Autodesk Fusion 360 part; units mm, degrees
(part 3 of 11)
  line L1668 (14.4479, -219.9183) -> (14.483, -219.9371)
  arc A104 (18.4614, -173.1211) -> (18.12, -173.2625) centre (18.32, -173.2625) ccw
  arc A105 (13.1828, -218.1997) -> (13.0414, -218.5411) centre (13.1828, -218.3997) ccw
  line L1669 (0.0013, -74.5276) -> (-0.0174, -74.5626)
  line L1670 (18.12, -173.2625) -> (18.12, -175.4997)
  line L1671 (6.2199, -29.9997) -> (6.02, -30.1995)
  line L1672 (-0.0787, -74.7914) -> (-0.08, -74.8997)
  line L1673 (0.0706, -74.4308) -> (0.0454, -74.4616)
  line L1674 (6.02, -29.7998) -> (6.2199, -29.9997)
  line L1675 (19.9148, -174.7519) -> (19.9083, -174.7127)
  line L1676 (-0.08, -74.8997) -> (-0.08, -78.4997)
  line L1677 (0.0454, -74.4616) -> (0.0223, -74.4938)
  line L1678 (-0.0338, -34.5988) -> (-0.0478, -34.636)
  line L1679 (14.3819, -219.8742) -> (14.4142, -219.8974)
  line L1680 (19.8738, -174.5988) -> (19.8574, -174.5626)
  line L1681 (6.02, -27.1603) -> (6.02, -29.7998)
  line L1682 (-0.0478, -74.636) -> (-0.0593, -74.674)
  line L1683 (19.8993, -174.674) -> (19.8878, -174.636)
  line L1684 (14.5943, -219.979) -> (14.633, -219.988)
  line L1685 (19.7946, -174.4616) -> (19.7694, -174.4308)
  line L1686 (14.3512, -219.849) -> (14.3819, -219.8742)
  line L1687 (6.02, -30.1995) -> (6.02, -32.839)
  line L1688 (-0.0683, -74.7127) -> (-0.0748, -74.7519)
  line L1689 (18.12, -175.4997) -> (16.4807, -175.4997)
  line L1690 (16.4807, -175.4997) -> (13.82, -172.839)
  line L1691 (3.6807, -37.2997) -> (7.0807, -33.8997)
  line L1692 (16.1593, -162.6997) -> (12.7593, -166.0997)
  line L1693 (7.0807, -173.8997) -> (9.713, -173.8997)
  line L1694 (9.92, -33.6927) -> (10.127, -33.8997)
  circle A106 centre (9.92, -29.9997) radius 2.1
  line L1695 (19.8177, -214.4938) -> (19.7946, -214.4616)
  arc A107 (1.72, -73.2625) -> (1.3786, -73.1211) centre (1.52, -73.2625) ccw
  line L1696 (18.12, -215.4997) -> (16.4807, -215.4997)
  line L1697 (-0.0593, -74.674) -> (-0.0683, -74.7127)
  arc A108 (1.72, -73.2625) -> (1.3786, -73.1211) centre (1.52, -73.2625) ccw
  line L1698 (19.8387, -214.5276) -> (19.8177, -214.4938)
  line L1699 (-0.0338, -74.5988) -> (-0.0478, -74.636)
  line L1700 (-0.0478, -74.636) -> (-0.0593, -74.674)
  line L1701 (14.483, -219.9371) -> (14.5191, -219.9534)
  line L1702 (16.1593, -162.6997) -> (12.7593, -166.0997)
  line L1703 (13.82, -167.1603) -> (16.4807, -164.4997)
  line L1704 (9.713, -166.0997) -> (7.0807, -166.0997)
  line L1705 (19.8387, -174.5276) -> (19.8177, -174.4938)
  line L1706 (16.4807, -175.4997) -> (13.82, -172.839)
  line L1707 (9.713, -33.8997) -> (9.92, -33.6927)
  line L1708 (9.713, -166.0997) -> (7.0807, -166.0997)
  line L1709 (18.42, -219.9997) -> (19.42, -219.9997)
  line L1710 (6.02, -32.839) -> (3.3593, -35.4997)
  line L1711 (-0.0174, -74.5626) -> (-0.0338, -74.5988)
  line L1712 (3.6807, -37.2997) -> (7.0807, -33.8997)
  line L1713 (0.0454, -74.4616) -> (0.0223, -74.4938)
  line L1714 (1.72, -35.4997) -> (1.72, -33.2625)
  line L1715 (-0.0338, -74.5988) -> (-0.0478, -74.636)
  line L1716 (0.0706, -74.4308) -> (0.0454, -74.4616)
  line L1717 (19.9187, -214.7914) -> (19.9148, -214.7519)
  line L1718 (3.3593, -75.4997) -> (1.72, -75.4997)
  line L1719 (6.02, -32.839) -> (3.3593, -35.4997)
  line L1720 (15.42, -218.1997) -> (13.1828, -218.1997)
  line L1721 (19.9148, -174.7519) -> (19.9083, -174.7127)
  line L1722 (-0.0174, -74.5626) -> (-0.0338, -74.5988)
  line L1723 (-0.0683, -74.7127) -> (-0.0748, -74.7519)
  line L1724 (13.82, -167.1603) -> (16.4807, -164.4997)
  line L1725 (19.8574, -174.5626) -> (19.8387, -174.5276)
  line L1726 (-0.08, -74.8997) -> (-0.08, -78.4997)
  line L1727 (9.92, -33.6927) -> (10.127, -33.8997)
  line L1728 (13.82, -30.1995) -> (13.6201, -29.9997)
  line L1729 (6.02, -72.839) -> (3.3593, -75.4997)
  line L1730 (4.42, -78.1997) -> (4.42, -76.5603)
  line L1731 (13.82, -32.839) -> (13.82, -30.1995)
  line L1732 (7.0807, -173.8997) -> (9.713, -173.8997)
  line L1733 (19.9083, -174.7127) -> (19.8993, -174.674)
  line L1734 (15.42, -216.5603) -> (15.42, -218.1997)
  line L1735 (1.72, -75.4997) -> (1.72, -73.2625)
  line L1736 (13.82, -29.7998) -> (13.82, -27.1603)
  arc A109 (6.7986, -78.5411) -> (6.6572, -78.1997) centre (6.6572, -78.3997) ccw
  line L1737 (19.9083, -214.7127) -> (19.8993, -214.674)
  line L1738 (13.0414, -218.5411) -> (14.3222, -219.8219)
  line L1739 (0.0223, -74.4938) -> (0.0013, -74.5276)
  line L1740 (1.72, -35.4997) -> (1.72, -33.2625)
  line L1741 (-0.0748, -74.7519) -> (-0.0787, -74.7914)
  line L1742 (0.0978, -74.4019) -> (0.0706, -74.4308)
  line L1743 (14.483, -219.9371) -> (14.5191, -219.9534)
  line L1744 (10.127, -33.8997) -> (12.7593, -33.8997)
  line L1745 (6.02, -72.839) -> (3.3593, -75.4997)
  line L1746 (13.6201, -29.9997) -> (13.82, -29.7998)
  line L1747 (13.82, -30.1995) -> (13.6201, -29.9997)
  line L1748 (4.42, -76.5603) -> (7.0807, -73.8997)
  line L1749 (13.82, -32.839) -> (13.82, -30.1995)
  line L1750 (19.8878, -214.636) -> (19.8738, -214.5988)
  line L1751 (13.6201, -29.9997) -> (13.82, -29.7998)
  line L1752 (1.3786, -73.1211) -> (0.0978, -74.4019)
  line L1753 (-0.08, -78.4997) -> (-0.08, -79.4997)
  line L1754 (19.8738, -214.5988) -> (19.8574, -214.5626)
  line L1755 (19.7694, -214.4308) -> (19.7422, -214.4019)
  arc A110 (13.0414, -81.4582) -> (13.1828, -81.7997) centre (13.1828, -81.5997) ccw
  line L1756 (19.92, -214.8311) -> (19.9187, -214.7914)
  line L1757 (9.7152, -73.8997) -> (9.92, -73.6949)
  line L1758 (19.7694, -34.4308) -> (19.7422, -34.4019)
  line L1759 (-0.08, -78.4997) -> (-0.08, -79.4997)
  line L1760 (19.92, -214.8311) -> (19.9187, -214.7914)
  line L1761 (10.127, -73.8997) -> (12.7593, -73.8997)
  line L1762 (19.7946, -214.4616) -> (19.7694, -214.4308)
  line L1763 (19.8574, -214.5626) -> (19.8387, -214.5276)
  line L1764 (18.12, -35.4997) -> (16.4807, -35.4997)
  line L1765 (4.42, -76.5603) -> (7.0807, -73.8997)
  arc A111 (19.42, -219.9997) -> (19.92, -219.4997) centre (19.42, -219.4997) ccw
  line L1766 (19.92, -219.4997) -> (19.92, -218.4997)
  line L1767 (4.42, -78.1997) -> (4.42, -76.5603)
  line L1768 (19.92, -218.4997) -> (19.92, -214.8311)
  line L1769 (5.5178, -79.8219) -> (6.7986, -78.5411)
  line L1770 (19.9083, -214.7127) -> (19.8993, -214.674)
  line L1771 (19.8574, -214.5626) -> (19.8387, -214.5276)
  line L1772 (19.7946, -214.4616) -> (19.7694, -214.4308)
  line L1773 (9.92, -73.6949) -> (10.127, -73.8997)
  line L1774 (18.12, -37.2997) -> (18.12, -42.6997)
  line L1775 (6.6572, -78.1997) -> (4.42, -78.1997)
  line L1776 (19.7694, -214.4308) -> (19.7422, -214.4019)
  line L1777 (19.8738, -34.5988) -> (19.8574, -34.5626)
  line L1778 (18.42, -219.9997) -> (19.42, -219.9997)
  arc A112 (19.42, -219.9997) -> (19.92, -219.4997) centre (19.42, -219.4997) ccw
  line L1779 (19.9148, -214.7519) -> (19.9083, -214.7127)
  line L1780 (5.5178, -79.8219) -> (6.7986, -78.5411)
  line L1781 (10.127, -33.8997) -> (12.7593, -33.8997)
  line L1782 (19.8177, -214.4938) -> (19.7946, -214.4616)
  line L1783 (19.92, -218.4997) -> (19.92, -214.8311)
  line L1784 (19.8387, -214.5276) -> (19.8177, -214.4938)
  line L1785 (9.713, -33.8997) -> (9.92, -33.6927)
  line L1786 (1.72, -75.4997) -> (1.72, -73.2625)
  line L1787 (19.8993, -214.674) -> (19.8878, -214.636)
  circle A113 centre (9.92, -29.9997) radius 2.1
  line L1788 (10.127, -73.8997) -> (12.7593, -73.8997)
  line L1789 (13.82, -29.7998) -> (13.82, -27.1603)
  line L1790 (9.92, -73.6949) -> (10.127, -73.8997)
  line L1791 (6.6572, -78.1997) -> (4.42, -78.1997)
  line L1792 (3.3593, -75.4997) -> (1.72, -75.4997)
  line L1793 (18.12, -42.6997) -> (16.1593, -42.6997)
  line L1794 (18.12, -33.2625) -> (18.12, -35.4997)
  line L1795 (19.9083, -34.7127) -> (19.8993, -34.674)
  line L1796 (19.92, -219.4997) -> (19.92, -218.4997)
  arc A114 (6.7986, -78.5411) -> (6.6572, -78.1997) centre (6.6572, -78.3997) ccw
  line L1797 (9.7152, -73.8997) -> (9.92, -73.6949)
  line L1798 (18.12, -215.4997) -> (16.4807, -215.4997)
  arc A115 (13.1828, -78.1997) -> (13.0414, -78.5411) centre (13.1828, -78.3997) ccw
  line L1799 (19.92, -34.8997) -> (19.9187, -34.7914)
  line L1800 (1.3786, -73.1211) -> (0.0978, -74.4019)
  line L1801 (19.9187, -214.7914) -> (19.9148, -214.7519)
  arc A116 (18.4614, -33.1211) -> (18.12, -33.2625) centre (18.32, -33.2625) ccw
  line L1802 (19.8993, -214.674) -> (19.8878, -214.636)
  arc A117 (13.1828, -78.1997) -> (13.0414, -78.5411) centre (13.1828, -78.3997) ccw
  arc A118 (13.0414, -81.4582) -> (13.1828, -81.7997) centre (13.1828, -81.5997) ccw
  line L1803 (19.8738, -214.5988) -> (19.8574, -214.5626)
  line L1804 (19.9083, -34.7127) -> (19.8993, -34.674)
  line L1805 (19.8878, -214.636) -> (19.8738, -214.5988)
  line L1806 (16.1593, -37.2997) -> (18.12, -37.2997)
  line L1807 (19.8574, -34.5626) -> (19.8387, -34.5276)
  line L1808 (19.7422, -214.4019) -> (18.4614, -213.1211)
  line L1809 (14.7514, -219.9997) -> (18.42, -219.9997)
  line L1810 (19.9148, -214.7519) -> (19.9083, -214.7127)
  line L1811 (18.12, -213.2625) -> (18.12, -215.4997)
  line L1812 (16.4807, -215.4997) -> (13.82, -212.839)
  line L1813 (19.8177, -34.4938) -> (19.7946, -34.4616)
  line L1814 (19.8738, -34.5988) -> (19.8574, -34.5626)
  line L1815 (12.7593, -213.8997) -> (15.42, -216.5603)
  line L1816 (18.12, -42.6997) -> (16.1593, -42.6997)
  line L1817 (14.7514, -219.9997) -> (18.42, -219.9997)
  line L1818 (-0.0787, -5.2079) -> (-0.0748, -5.2474)
  line L1819 (0.0978, -5.5975) -> (1.3786, -6.8782)
  line L1820 (5.2457, -0.0203) -> (5.207, -0.0113)
  line L1821 (4.42, -3.439) -> (4.42, -1.7997)
  line L1822 (5.207, -0.0113) -> (5.1678, -0.0049)
  line L1823 (5.4888, -0.1503) -> (5.4581, -0.1251)
  line L1824 (4.42, -1.7997) -> (6.6572, -1.7997)
  line L1825 (-0.08, -1.4997) -> (-0.08, -5.0997)
  line L1826 (1.42, 0.0003) -> (0.42, 0.0003)
  arc A119 (6.6572, -1.7997) -> (6.7986, -1.4582) centre (6.6572, -1.5997) ccw
  line L1827 (1.72, -4.4997) -> (3.3593, -4.4997)
  line L1828 (-0.0787, -5.2079) -> (-0.0748, -5.2474)
  line L1829 (7.0807, -6.0997) -> (4.42, -3.439)
  line L1830 (5.357, -0.0623) -> (5.3209, -0.0459)
  line L1831 (5.1283, -0.001) -> (5.0886, 0.0003)
  line L1832 (5.0886, 0.0003) -> (1.42, 0.0003)
  line L1833 (5.4258, -0.102) -> (5.3921, -0.081)
  arc A120 (13.0414, -1.4582) -> (13.1828, -1.7997) centre (13.1828, -1.5997) ccw
  line L1834 (13.6201, -9.9997) -> (13.82, -9.7998)
  line L1835 (-0.08, -1.4997) -> (-0.08, -5.0997)
  line L1836 (9.92, -6.3044) -> (9.7152, -6.0997)
  line L1837 (6.7986, -1.4582) -> (5.5178, -0.1775)
  line L1838 (12.7593, -6.0997) -> (10.127, -6.0997)
  line L1839 (7.0807, -6.0997) -> (4.42, -3.439)
  line L1840 (-0.0683, -5.2866) -> (-0.0593, -5.3253)
  line L1841 (1.42, 0.0003) -> (0.42, 0.0003)
  line L1842 (9.92, -6.3044) -> (9.7152, -6.0997)
  line L1843 (5.2837, -0.0319) -> (5.2457, -0.0203)
  line L1844 (5.4581, -0.1251) -> (5.4258, -0.102)
  line L1845 (5.2457, -0.0203) -> (5.207, -0.0113)
  line L1846 (-0.08, -0.4997) -> (-0.08, -1.4997)
  line L1847 (3.3593, -4.4997) -> (6.02, -7.1603)
  line L1848 (5.207, -0.0113) -> (5.1678, -0.0049)
  arc A121 (0.42, 0.0003) -> (-0.08, -0.4997) centre (0.42, -0.4997) ccw
  line L1849 (5.5178, -0.1775) -> (5.4888, -0.1503)
  line L1850 (5.1678, -0.0049) -> (5.1283, -0.001)
  line L1851 (1.72, -6.7368) -> (1.72, -4.4997)
  line L1852 (5.4258, -0.102) -> (5.3921, -0.081)
  line L1853 (1.72, -6.7368) -> (1.72, -4.4997)
  line L1854 (-0.08, -0.4997) -> (-0.08, -1.4997)
  line L1855 (5.3921, -0.081) -> (5.357, -0.0623)
  line L1856 (3.3593, -4.4997) -> (6.02, -7.1603)
  arc A122 (0.42, 0.0003) -> (-0.08, -0.4997) centre (0.42, -0.4997) ccw
  line L1857 (-0.0593, -5.3253) -> (-0.0478, -5.3633)
  line L1858 (5.5178, -0.1775) -> (5.4888, -0.1503)
  line L1859 (4.42, -3.439) -> (4.42, -1.7997)
  line L1860 (5.2837, -0.0319) -> (5.2457, -0.0203)
  line L1861 (6.7986, -1.4582) -> (5.5178, -0.1775)
  line L1862 (5.3921, -0.081) -> (5.357, -0.0623)
  line L1863 (0.0454, -5.5378) -> (0.0706, -5.5685)
  line L1864 (0.0706, -5.5685) -> (0.0978, -5.5975)
  line L1865 (5.3209, -0.0459) -> (5.2837, -0.0319)
  arc A123 (6.6572, -1.7997) -> (6.7986, -1.4582) centre (6.6572, -1.5997) ccw
  line L1866 (5.3209, -0.0459) -> (5.2837, -0.0319)
  line L1867 (5.357, -0.0623) -> (5.3209, -0.0459)
  line L1868 (5.1678, -0.0049) -> (5.1283, -0.001)
  line L1869 (5.4581, -0.1251) -> (5.4258, -0.102)
  line L1870 (-0.08, -5.0997) -> (-0.0787, -5.2079)
  line L1871 (0.0978, -5.5975) -> (1.3786, -6.8782)
  line L1872 (5.0886, 0.0003) -> (1.42, 0.0003)
  line L1873 (5.4888, -0.1503) -> (5.4581, -0.1251)
  line L1874 (0.0978, -25.5975) -> (1.3786, -26.8782)
  line L1875 (5.1283, -0.001) -> (5.0886, 0.0003)
  line L1876 (4.42, -1.7997) -> (6.6572, -1.7997)
  line L1877 (14.7117, -80.001) -> (14.6722, -80.0049)
  line L1878 (7.0807, -33.8997) -> (9.713, -33.8997)
  arc A124 (19.42, -79.9997) -> (19.92, -79.4997) centre (19.42, -79.4997) ccw
  line L1879 (0.0223, -25.5055) -> (0.0454, -25.5378)
  line L1880 (14.5563, -80.0319) -> (14.5191, -80.0459)
  line L1881 (-0.08, -34.8997) -> (-0.08, -45.0997)
  line L1882 (19.92, -45.0997) -> (19.92, -34.8997)
  line L1883 (-0.0593, -25.3253) -> (-0.0478, -25.3633)
  line L1884 (14.633, -80.0113) -> (14.5943, -80.0203)
  line L1885 (7.0807, -46.0997) -> (3.6807, -42.6997)
  line L1886 (-0.0787, -25.2079) -> (-0.0748, -25.2474)
  line L1887 (14.633, -80.0113) -> (14.5943, -80.0203)
  line L1888 (19.92, -81.4997) -> (19.92, -80.4997)
  line L1889 (14.7117, -79.9984) -> (14.7514, -79.9997)
  line L1890 (14.633, -79.988) -> (14.6722, -79.9945)
  line L1891 (14.6722, -80.0049) -> (14.633, -80.0113)
  line L1892 (18.42, -79.9997) -> (19.42, -79.9997)
  arc A125 (19.92, -80.4997) -> (19.42, -79.9997) centre (19.42, -80.4997) ccw
  line L1893 (14.5943, -80.0203) -> (14.5563, -80.0319)
  line L1894 (1.72, -26.7368) -> (1.72, -24.4997)
  line L1895 (-0.0683, -25.2866) -> (-0.0593, -25.3253)
  line L1896 (18.42, -79.9997) -> (14.7514, -79.9997)
  line L1897 (14.5563, -79.9674) -> (14.5943, -79.979)
  line L1898 (14.6722, -79.9945) -> (14.7117, -79.9984)
  arc A126 (19.42, -79.9997) -> (19.92, -79.4997) centre (19.42, -79.4997) ccw
  line L1899 (14.5943, -79.979) -> (14.633, -79.988)
  line L1900 (14.7117, -79.9984) -> (14.7514, -79.9997)
  line L1901 (14.6722, -80.0049) -> (14.633, -80.0113)
  line L1902 (14.5191, -79.9534) -> (14.5563, -79.9674)
  line L1903 (14.7514, -79.9997) -> (18.42, -79.9997)
  line L1904 (0.0223, -25.5055) -> (0.0454, -25.5378)
  line L1905 (18.12, -75.4997) -> (16.4807, -75.4997)
  line L1906 (0.0013, -25.4717) -> (0.0223, -25.5055)
  line L1907 (14.5563, -79.9674) -> (14.5943, -79.979)
  line L1908 (7.0807, -46.0997) -> (3.6807, -42.6997)
  line L1909 (16.1593, -42.6997) -> (12.7593, -46.0997)
  line L1910 (0.0454, -25.5378) -> (0.0706, -25.5685)
  line L1911 (19.42, -79.9997) -> (18.42, -79.9997)
  line L1912 (14.7117, -80.001) -> (14.6722, -80.0049)
  line L1913 (14.5563, -80.0319) -> (14.5191, -80.0459)
  line L1914 (16.1593, -42.6997) -> (12.7593, -46.0997)
  line L1915 (14.633, -79.988) -> (14.6722, -79.9945)
  arc A127 (19.92, -80.4997) -> (19.42, -79.9997) centre (19.42, -80.4997) ccw
  line L1916 (14.7514, -79.9997) -> (14.7117, -80.001)
  line L1917 (14.7514, -79.9997) -> (18.42, -79.9997)
  line L1918 (-0.0338, -25.4005) -> (-0.0174, -25.4367)
  line L1919 (0.0013, -25.4717) -> (0.0223, -25.5055)
  line L1920 (14.5943, -79.979) -> (14.633, -79.988)
  line L1921 (-0.0338, -25.4005) -> (-0.0174, -25.4367)
  line L1922 (19.92, -45.0997) -> (19.92, -34.8997)
  line L1923 (-0.0174, -25.4367) -> (0.0013, -25.4717)
  line L1924 (19.92, -81.4997) -> (19.92, -80.4997)
  line L1925 (-0.08, -34.8997) -> (-0.08, -45.0997)
  line L1926 (14.5943, -80.0203) -> (14.5563, -80.0319)
  line L1927 (14.6722, -79.9945) -> (14.7117, -79.9984)
  line L1928 (14.5191, -79.9534) -> (14.5563, -79.9674)
  line L1929 (18.42, -79.9997) -> (19.42, -79.9997)
  line L1930 (14.7514, -79.9997) -> (14.7117, -80.001)
  line L1931 (19.42, -79.9997) -> (18.42, -79.9997)
  line L1932 (-0.08, -25.0997) -> (-0.0787, -25.2079)
  line L1933 (18.42, -79.9997) -> (14.7514, -79.9997)
  line L1934 (-0.0748, -25.2474) -> (-0.0683, -25.2866)
  line L1935 (15.42, -76.5603) -> (15.42, -78.1997)
  line L1936 (0.0706, -25.5685) -> (0.0978, -25.5975)
  line L1937 (-0.0683, -14.7127) -> (-0.0748, -14.7519)
  line L1938 (0.0706, -25.5685) -> (0.0978, -25.5975)
  line L1939 (19.8387, -74.5276) -> (19.8177, -74.4938)
  arc A128 (18.4614, -73.1211) -> (18.12, -73.2625) centre (18.32, -73.2625) ccw
  line L1940 (0.0454, -14.4616) -> (0.0223, -14.4938)
  line L1941 (19.9083, -74.7127) -> (19.8993, -74.674)
  line L1942 (19.9148, -74.7519) -> (19.9083, -74.7127)
  line L1943 (-0.0787, -14.7914) -> (-0.08, -14.8997)
  line L1944 (19.8177, -74.4938) -> (19.7946, -74.4616)
  line L1945 (0.0454, -25.5378) -> (0.0706, -25.5685)
  line L1946 (1.72, -26.7368) -> (1.72, -24.4997)
  line L1947 (19.8387, -74.5276) -> (19.8177, -74.4938)
  line L1948 (19.92, -78.4997) -> (19.92, -74.8311)
  line L1949 (19.8574, -74.5626) -> (19.8387, -74.5276)
  line L1950 (19.7694, -74.4308) -> (19.7422, -74.4019)
  line L1951 (18.12, -73.2625) -> (18.12, -75.4997)
  line L1952 (19.7946, -74.4616) -> (19.7694, -74.4308)
  line L1953 (-0.0787, -25.2079) -> (-0.0748, -25.2474)
  line L1954 (19.8177, -74.4938) -> (19.7946, -74.4616)
  line L1955 (18.12, -75.4997) -> (16.4807, -75.4997)
  line L1956 (19.8738, -74.5988) -> (19.8574, -74.5626)
  line L1957 (19.8993, -74.674) -> (19.8878, -74.636)
  line L1958 (-0.08, -25.0997) -> (-0.0787, -25.2079)
  line L1959 (0.0978, -14.4019) -> (0.0706, -14.4308)
  line L1960 (-0.0338, -14.5988) -> (-0.0478, -14.636)
  line L1961 (15.42, -76.5603) -> (15.42, -78.1997)
  line L1962 (-0.0174, -25.4367) -> (0.0013, -25.4717)
  line L1963 (-0.0748, -25.2474) -> (-0.0683, -25.2866)
  line L1964 (-0.0683, -25.2866) -> (-0.0593, -25.3253)
  line L1965 (1.72, -22.6997) -> (1.72, -17.2997)
  line L1966 (18.12, -73.2625) -> (18.12, -75.4997)
  line L1967 (19.92, -78.4997) -> (19.92, -74.8311)
  line L1968 (-0.0478, -25.3633) -> (-0.0338, -25.4005)
  line L1969 (-0.0478, -25.3633) -> (-0.0338, -25.4005)
  line L1970 (0.0013, -14.5276) -> (-0.0174, -14.5626)
  line L1971 (19.8878, -74.636) -> (19.8738, -74.5988)
  line L1972 (-0.0478, -14.636) -> (-0.0593, -14.674)
  line L1973 (19.8993, -74.674) -> (19.8878, -74.636)
  arc A129 (1.72, -13.2625) -> (1.3786, -13.1211) centre (1.52, -13.2625) ccw
  line L1974 (19.7946, -74.4616) -> (19.7694, -74.4308)
  line L1975 (-0.0787, -14.7914) -> (-0.08, -14.8997)
  line L1976 (1.72, -15.4997) -> (1.72, -13.2625)
  line L1977 (19.8738, -74.5988) -> (19.8574, -74.5626)
  line L1978 (19.8878, -74.636) -> (19.8738, -74.5988)
  line L1979 (0.0223, -14.4938) -> (0.0013, -14.5276)
  line L1980 (19.7694, -74.4308) -> (19.7422, -74.4019)
  line L1981 (19.92, -74.8311) -> (19.9187, -74.7914)
  line L1982 (0.0706, -14.4308) -> (0.0454, -14.4616)
  line L1983 (19.92, -74.8311) -> (19.9187, -74.7914)
  line L1984 (19.9187, -74.7914) -> (19.9148, -74.7519)
  line L1985 (19.7422, -74.4019) -> (18.4614, -73.1211)
  line L1986 (19.9083, -74.7127) -> (19.8993, -74.674)
  line L1987 (-0.0593, -25.3253) -> (-0.0478, -25.3633)
  arc A130 (18.4614, -73.1211) -> (18.12, -73.2625) centre (18.32, -73.2625) ccw
  line L1988 (19.9187, -74.7914) -> (19.9148, -74.7519)
  line L1989 (19.8574, -74.5626) -> (19.8387, -74.5276)
  line L1990 (0.0013, -14.5276) -> (-0.0174, -14.5626)
  line L1991 (19.9148, -74.7519) -> (19.9083, -74.7127)
  line L1992 (19.7422, -74.4019) -> (18.4614, -73.1211)
  line L1993 (1.3786, -13.1211) -> (0.0978, -14.4019)
  line L1994 (19.92, -79.4997) -> (19.92, -78.4997)
  line L1995 (-0.0174, -14.5626) -> (-0.0338, -14.5988)
  line L1996 (1.72, -22.6997) -> (1.72, -17.2997)
  line L1997 (19.92, -79.4997) -> (19.92, -78.4997)
  line L1998 (0.0223, -14.4938) -> (0.0013, -14.5276)
  line L1999 (10.127, -13.8997) -> (12.7593, -13.8997)
  line L2000 (9.92, -26.3066) -> (9.713, -26.0997)
  line L2001 (10.127, -13.8997) -> (12.7593, -13.8997)
  line L2002 (6.02, -12.839) -> (3.3593, -15.4997)
  line L2003 (7.0807, -73.8997) -> (9.7152, -73.8997)
  arc A131 (1.3786, -66.8782) -> (1.72, -66.7368) centre (1.52, -66.7368) ccw
  line L2004 (-0.0683, -65.2866) -> (-0.0593, -65.3253)
  line L2005 (10.127, -26.0997) -> (9.92, -26.3066)
  line L2006 (-0.0338, -65.4005) -> (-0.0174, -65.4367)
  line L2007 (0.0978, -65.5975) -> (1.3786, -66.8782)
  line L2008 (9.713, -13.8997) -> (9.92, -13.6927)
  line L2009 (-0.0593, -65.3253) -> (-0.0478, -65.3633)
  line L2010 (13.1828, -81.7997) -> (15.42, -81.7997)
  line L2011 (-0.0338, -14.5988) -> (-0.0478, -14.636)
  line L2012 (-0.0748, -14.7519) -> (-0.0787, -14.7914)
  line L2013 (6.2199, -69.9997) -> (6.02, -70.1995)
  line L2014 (-0.0683, -14.7127) -> (-0.0748, -14.7519)
  line L2015 (13.1828, -81.7997) -> (15.42, -81.7997)
  line L2016 (-0.0174, -65.4367) -> (0.0013, -65.4717)
  line L2017 (6.02, -69.7998) -> (6.2199, -69.9997)
  line L2018 (9.92, -26.3066) -> (9.713, -26.0997)
  line L2019 (9.713, -26.0997) -> (7.0807, -26.0997)
  line L2020 (3.6807, -17.2997) -> (7.0807, -13.8997)
  line L2021 (0.0454, -14.4616) -> (0.0223, -14.4938)
  line L2022 (7.0807, -26.0997) -> (3.6807, -22.6997)
  line L2023 (0.0454, -65.5378) -> (0.0706, -65.5685)
  line L2024 (13.0414, -78.5411) -> (14.3222, -79.8219)
  line L2025 (-0.08, -14.8997) -> (-0.08, -25.0997)
  line L2026 (16.4807, -75.4997) -> (13.82, -72.839)
  line L2027 (12.7593, -73.8997) -> (15.42, -76.5603)
  line L2028 (6.2199, -69.9997) -> (6.02, -70.1995)
  line L2029 (14.3222, -80.1775) -> (13.0414, -81.4582)
  line L2030 (-0.0174, -14.5626) -> (-0.0338, -14.5988)
  line L2031 (6.02, -12.839) -> (3.3593, -15.4997)
  line L2032 (16.4807, -75.4997) -> (13.82, -72.839)
  line L2033 (-0.0478, -14.636) -> (-0.0593, -14.674)
  line L2034 (1.72, -15.4997) -> (1.72, -13.2625)
  line L2035 (15.42, -78.1997) -> (13.1828, -78.1997)
  line L2036 (-0.0593, -14.674) -> (-0.0683, -14.7127)
  line L2037 (-0.0748, -14.7519) -> (-0.0787, -14.7914)
  line L2038 (-0.08, -14.8997) -> (-0.08, -25.0997)
  line L2039 (0.0706, -14.4308) -> (0.0454, -14.4616)
  line L2040 (13.82, -72.839) -> (13.82, -70.1995)
  line L2041 (6.02, -69.7998) -> (6.2199, -69.9997)
  line L2042 (7.0807, -73.8997) -> (9.7152, -73.8997)
  line L2043 (7.0807, -13.8997) -> (9.713, -13.8997)
  line L2044 (9.92, -13.6927) -> (10.127, -13.8997)
  line L2045 (0.0223, -65.5055) -> (0.0454, -65.5378)
  line L2046 (14.3222, -80.1775) -> (13.0414, -81.4582)
  arc A132 (1.72, -13.2625) -> (1.3786, -13.1211) centre (1.52, -13.2625) ccw
  line L2047 (1.3786, -13.1211) -> (0.0978, -14.4019)
  line L2048 (0.0978, -14.4019) -> (0.0706, -14.4308)
  line L2049 (12.7593, -73.8997) -> (15.42, -76.5603)
  line L2050 (13.0414, -78.5411) -> (14.3222, -79.8219)
  line L2051 (-0.0593, -14.674) -> (-0.0683, -14.7127)
  line L2052 (7.0807, -26.0997) -> (3.6807, -22.6997)
  line L2053 (15.42, -78.1997) -> (13.1828, -78.1997)
  line L2054 (12.7593, -26.0997) -> (10.127, -26.0997)
  arc A133 (1.3786, -66.8782) -> (1.72, -66.7368) centre (1.52, -66.7368) ccw
  line L2055 (0.0706, -65.5685) -> (0.0978, -65.5975)
  line L2056 (0.0013, -65.4717) -> (0.0223, -65.5055)
  line L2057 (-0.0748, -65.2474) -> (-0.0683, -65.2866)
  line L2058 (12.7593, -26.0997) -> (10.127, -26.0997)
  line L2059 (3.6807, -17.2997) -> (7.0807, -13.8997)
  line L2060 (0.0013, -65.4717) -> (0.0223, -65.5055)
  line L2061 (9.92, -66.3066) -> (9.713, -66.0997)
  line L2062 (13.6201, -69.9997) -> (13.82, -69.7998)
  line L2063 (19.9083, -25.2866) -> (19.9148, -25.2474)
  line L2064 (19.8387, -25.4717) -> (19.8574, -25.4367)
  line L2065 (10.127, -66.0997) -> (9.92, -66.3066)
  line L2066 (1.72, -64.4997) -> (3.3593, -64.4997)
  line L2067 (-0.0748, -65.2474) -> (-0.0683, -65.2866)
  line L2068 (10.127, -26.0997) -> (9.92, -26.3066)
  line L2069 (0.0223, -65.5055) -> (0.0454, -65.5378)
  line L2070 (9.92, -13.6927) -> (10.127, -13.8997)
  line L2071 (-0.0174, -65.4367) -> (0.0013, -65.4717)
  line L2072 (-0.0787, -65.2079) -> (-0.0748, -65.2474)
  line L2073 (-0.0478, -65.3633) -> (-0.0338, -65.4005)
  line L2074 (-0.0787, -65.2079) -> (-0.0748, -65.2474)
  line L2075 (-0.0593, -65.3253) -> (-0.0478, -65.3633)
  line L2076 (1.72, -24.4997) -> (3.3593, -24.4997)
  line L2077 (0.0978, -65.5975) -> (1.3786, -66.8782)
  line L2078 (1.72, -64.4997) -> (3.3593, -64.4997)
  line L2079 (7.0807, -66.0997) -> (3.6807, -62.6997)
  line L2080 (19.8574, -25.4367) -> (19.8738, -25.4005)
  line L2081 (19.8993, -25.3253) -> (19.9083, -25.2866)
  line L2082 (19.9187, -25.2079) -> (19.92, -25.0997)
  line L2083 (9.713, -13.8997) -> (9.92, -13.6927)
  line L2084 (-0.0683, -65.2866) -> (-0.0593, -65.3253)
  line L2085 (-0.08, -65.0997) -> (-0.0787, -65.2079)
  line L2086 (16.4807, -24.4997) -> (18.12, -24.4997)
  line L2087 (3.6807, -22.6997) -> (1.72, -22.6997)
  line L2088 (3.3593, -15.4997) -> (1.72, -15.4997)
  line L2089 (-0.0478, -65.3633) -> (-0.0338, -65.4005)
  line L2090 (1.72, -17.2997) -> (3.6807, -17.2997)
  line L2091 (1.72, -24.4997) -> (3.3593, -24.4997)
  line L2092 (6.02, -67.1603) -> (6.02, -69.7998)
  line L2093 (3.6807, -62.6997) -> (1.72, -62.6997)
  line L2094 (3.6807, -62.6997) -> (1.72, -62.6997)
  line L2095 (3.3593, -64.4997) -> (6.02, -67.1603)
  line L2096 (0.0706, -65.5685) -> (0.0978, -65.5975)
  line L2097 (1.72, -66.7368) -> (1.72, -64.4997)
  line L2098 (1.72, -66.7368) -> (1.72, -64.4997)
  line L2099 (3.3593, -64.4997) -> (6.02, -67.1603)
  line L2100 (0.0454, -65.5378) -> (0.0706, -65.5685)
  line L2101 (3.6807, -22.6997) -> (1.72, -22.6997)
  line L2102 (7.0807, -66.0997) -> (3.6807, -62.6997)
  line L2103 (19.9148, -25.2474) -> (19.9187, -25.2079)
  line L2104 (-0.0338, -65.4005) -> (-0.0174, -65.4367)
  line L2105 (19.8738, -25.4005) -> (19.8878, -25.3633)
  line L2106 (18.12, -24.4997) -> (18.12, -26.7368)
  line L2107 (19.7422, -25.5975) -> (19.7694, -25.5685)
  line L2108 (10.127, -66.0997) -> (9.92, -66.3066)
  line L2109 (7.0807, -13.8997) -> (9.713, -13.8997)
  line L2110 (9.713, -26.0997) -> (7.0807, -26.0997)
  line L2111 (3.3593, -15.4997) -> (1.72, -15.4997)
  line L2112 (1.72, -17.2997) -> (3.6807, -17.2997)
  line L2113 (6.02, -67.1603) -> (6.02, -69.7998)
  line L2114 (19.7946, -25.5378) -> (19.8177, -25.5055)
  line L2115 (13.82, -69.7998) -> (13.82, -67.1603)
  line L2116 (13.6201, -69.9997) -> (13.82, -69.7998)
  line L2117 (19.8387, -25.4717) -> (19.8574, -25.4367)
  line L2118 (-0.08, -65.0997) -> (-0.0787, -65.2079)
  line L2119 (19.9148, -25.2474) -> (19.9187, -25.2079)
  line L2120 (19.9083, -25.2866) -> (19.9148, -25.2474)
  line L2121 (13.82, -69.7998) -> (13.82, -67.1603)
  line L2122 (19.7694, -25.5685) -> (19.7946, -25.5378)
  line L2123 (13.82, -27.1603) -> (16.4807, -24.4997)
  line L2124 (19.8574, -65.4367) -> (19.8738, -65.4005)
  line L2125 (19.8878, -65.3633) -> (19.8993, -65.3253)
  line L2126 (19.7694, -65.5685) -> (19.7946, -65.5378)
  line L2127 (18.12, -17.2997) -> (18.12, -22.6997)
  line L2128 (16.1593, -17.2997) -> (18.12, -17.2997)
  line L2129 (19.7946, -65.5378) -> (19.8177, -65.5055)
  line L2130 (18.4614, -66.8782) -> (19.7422, -65.5975)
  line L2131 (19.8387, -65.4717) -> (19.8574, -65.4367)
  line L2132 (18.12, -22.6997) -> (16.1593, -22.6997)
  line L2133 (19.8574, -25.4367) -> (19.8738, -25.4005)
  line L2134 (19.7694, -65.5685) -> (19.7946, -65.5378)
  line L2135 (19.8738, -65.4005) -> (19.8878, -65.3633)
  line L2136 (19.9083, -65.2866) -> (19.9148, -65.2474)
  arc A134 (18.4614, -13.1211) -> (18.12, -13.2625) centre (18.32, -13.2625) ccw
  line L2137 (19.8387, -65.4717) -> (19.8574, -65.4367)
  line L2138 (19.9083, -14.7127) -> (19.8993, -14.674)
  line L2139 (19.8177, -25.5055) -> (19.8387, -25.4717)
  line L2140 (19.7946, -25.5378) -> (19.8177, -25.5055)
  line L2141 (19.7694, -25.5685) -> (19.7946, -25.5378)
  line L2142 (19.9083, -65.2866) -> (19.9148, -65.2474)
  line L2143 (19.9148, -65.2474) -> (19.9187, -65.2079)
  line L2144 (19.8878, -25.3633) -> (19.8993, -25.3253)
  line L2145 (16.1593, -17.2997) -> (18.12, -17.2997)
  line L2146 (18.12, -17.2997) -> (18.12, -22.6997)
  line L2147 (19.8574, -65.4367) -> (19.8738, -65.4005)
  line L2148 (19.8738, -25.4005) -> (19.8878, -25.3633)
  line L2149 (18.4614, -66.8782) -> (19.7422, -65.5975)
  line L2150 (18.12, -62.6997) -> (16.1593, -62.6997)
  line L2151 (19.8177, -25.5055) -> (19.8387, -25.4717)
  line L2152 (19.7946, -14.4616) -> (19.7694, -14.4308)
  line L2153 (18.12, -64.4997) -> (18.12, -66.7368)
  arc A135 (18.12, -26.7368) -> (18.4614, -26.8782) centre (18.32, -26.7368) ccw
  line L2154 (12.7593, -66.0997) -> (10.127, -66.0997)
  line L2155 (19.9148, -65.2474) -> (19.9187, -65.2079)
  line L2156 (19.7422, -65.5975) -> (19.7694, -65.5685)
  line L2157 (16.4807, -24.4997) -> (18.12, -24.4997)
  line L2158 (9.92, -66.3066) -> (9.713, -66.0997)
  arc A136 (18.12, -66.7368) -> (18.4614, -66.8782) centre (18.32, -66.7368) ccw
  line L2159 (19.8177, -65.5055) -> (19.8387, -65.4717)
  line L2160 (19.8738, -65.4005) -> (19.8878, -65.3633)
  line L2161 (19.7422, -65.5975) -> (19.7694, -65.5685)
  line L2162 (13.82, -70.1995) -> (13.6201, -69.9997)
  line L2163 (13.82, -70.1995) -> (13.6201, -69.9997)
  line L2164 (18.12, -24.4997) -> (18.12, -26.7368)
  line L2165 (19.8993, -65.3253) -> (19.9083, -65.2866)
  line L2166 (19.8177, -65.5055) -> (19.8387, -65.4717)
  arc A137 (18.12, -66.7368) -> (18.4614, -66.8782) centre (18.32, -66.7368) ccw
  line L2167 (19.8993, -65.3253) -> (19.9083, -65.2866)
  line L2168 (18.12, -22.6997) -> (16.1593, -22.6997)
  line L2169 (16.4807, -64.4997) -> (18.12, -64.4997)
  line L2170 (18.12, -62.6997) -> (16.1593, -62.6997)
  line L2171 (16.4807, -64.4997) -> (18.12, -64.4997)
  line L2172 (18.12, -15.4997) -> (16.4807, -15.4997)
  line L2173 (19.7422, -25.5975) -> (19.7694, -25.5685)
  line L2174 (19.8878, -25.3633) -> (19.8993, -25.3253)
  line L2175 (19.9187, -25.2079) -> (19.92, -25.0997)
  line L2176 (19.8993, -25.3253) -> (19.9083, -25.2866)
  line L2177 (12.7593, -66.0997) -> (10.127, -66.0997)
  line L2178 (19.7946, -65.5378) -> (19.8177, -65.5055)
  line L2179 (19.8878, -65.3633) -> (19.8993, -65.3253)
  line L2180 (19.8738, -14.5988) -> (19.8574, -14.5626)
  line L2181 (19.9083, -14.7127) -> (19.8993, -14.674)
  line L2182 (18.12, -13.2625) -> (18.12, -15.4997)
  line L2183 (16.1593, -62.6997) -> (12.7593, -66.0997)
  line L2184 (13.82, -67.1603) -> (16.4807, -64.4997)
  line L2185 (19.8993, -14.674) -> (19.8878, -14.636)
  line L2186 (18.4614, -26.8782) -> (19.7422, -25.5975)
  line L2187 (12.7593, -13.8997) -> (16.1593, -17.2997)
  line L2188 (6.02, -70.1995) -> (6.02, -72.839)
  line L2189 (3.3593, -24.4997) -> (6.02, -27.1603)
  line L2190 (6.2199, -9.9997) -> (6.02, -10.1995)
  line L2191 (0.0454, -5.5378) -> (0.0706, -5.5685)
  line L2192 (0.0706, -5.5685) -> (0.0978, -5.5975)
  line L2193 (16.4807, -15.4997) -> (13.82, -12.839)
  line L2194 (19.9148, -14.7519) -> (19.9083, -14.7127)
  line L2195 (19.8574, -14.5626) -> (19.8387, -14.5276)
  line L2196 (19.7422, -14.4019) -> (18.4614, -13.1211)
  line L2197 (16.4807, -15.4997) -> (13.82, -12.839)
  line L2198 (19.9187, -65.2079) -> (19.92, -65.0997)
  arc A138 (18.4614, -13.1211) -> (18.12, -13.2625) centre (18.32, -13.2625) ccw
  line L2199 (19.7946, -14.4616) -> (19.7694, -14.4308)
  line L2200 (19.9187, -14.7914) -> (19.9148, -14.7519)
  line L2201 (19.8574, -14.5626) -> (19.8387, -14.5276)
  circle A139 centre (9.92, -69.9997) radius 2.1
  line L2202 (19.92, -25.0997) -> (19.92, -14.8997)
  line L2203 (12.7593, -13.8997) -> (16.1593, -17.2997)
  arc A140 (1.3786, -26.8782) -> (1.72, -26.7368) centre (1.52, -26.7368) ccw
  line L2204 (9.713, -66.0997) -> (7.0807, -66.0997)
  arc A141 (1.3786, -6.8782) -> (1.72, -6.7368) centre (1.52, -6.7368) ccw
  line L2205 (13.82, -72.839) -> (13.82, -70.1995)
  line L2206 (6.2199, -9.9997) -> (6.02, -10.1995)
  line L2207 (19.8387, -14.5276) -> (19.8177, -14.4938)
  line L2208 (19.9187, -14.7914) -> (19.9148, -14.7519)
  line L2209 (19.8387, -14.5276) -> (19.8177, -14.4938)
  line L2210 (19.7694, -14.4308) -> (19.7422, -14.4019)
  line L2211 (19.9187, -65.2079) -> (19.92, -65.0997)
  line L2212 (19.8738, -14.5988) -> (19.8574, -14.5626)
  line L2213 (6.02, -70.1995) -> (6.02, -72.839)
  line L2214 (19.9148, -14.7519) -> (19.9083, -14.7127)
  line L2215 (19.8993, -14.674) -> (19.8878, -14.636)
  line L2216 (18.12, -13.2625) -> (18.12, -15.4997)
  line L2217 (19.8878, -14.636) -> (19.8738, -14.5988)
  line L2218 (19.92, -25.0997) -> (19.92, -14.8997)
  line L2219 (16.1593, -22.6997) -> (12.7593, -26.0997)
  line L2220 (19.8177, -14.4938) -> (19.7946, -14.4616)
  line L2221 (6.02, -9.7998) -> (6.2199, -9.9997)
  line L2222 (16.1593, -22.6997) -> (12.7593, -26.0997)
  line L2223 (6.02, -7.1603) -> (6.02, -9.7998)
  line L2224 (13.82, -67.1603) -> (16.4807, -64.4997)
  line L2225 (19.8177, -14.4938) -> (19.7946, -14.4616)
  line L2226 (6.02, -9.7998) -> (6.2199, -9.9997)
  line L2227 (0.0223, -5.5055) -> (0.0454, -5.5378)
  line L2228 (0.0013, -5.4717) -> (0.0223, -5.5055)
  line L2229 (-0.08, -5.0997) -> (-0.0787, -5.2079)
  arc A142 (1.3786, -6.8782) -> (1.72, -6.7368) centre (1.52, -6.7368) ccw
  line L2230 (19.92, -14.8997) -> (19.9187, -14.7914)
  line L2231 (9.713, -66.0997) -> (7.0807, -66.0997)
  line L2232 (16.1593, -62.6997) -> (12.7593, -66.0997)
  line L2233 (19.8878, -14.636) -> (19.8738, -14.5988)
  circle A143 centre (9.92, -69.9997) radius 2.1
  line L2234 (18.12, -64.4997) -> (18.12, -66.7368)
  line L2235 (19.7694, -14.4308) -> (19.7422, -14.4019)
  line L2236 (19.92, -14.8997) -> (19.9187, -14.7914)
  line L2237 (19.7422, -14.4019) -> (18.4614, -13.1211)
  line L2238 (18.12, -15.4997) -> (16.4807, -15.4997)
  arc A144 (18.12, -26.7368) -> (18.4614, -26.8782) centre (18.32, -26.7368) ccw
  line L2239 (6.02, -7.1603) -> (6.02, -9.7998)
  line L2240 (-0.0748, -5.2474) -> (-0.0683, -5.2866)
  line L2241 (-0.0338, -5.4005) -> (-0.0174, -5.4367)
  line L2242 (1.72, -4.4997) -> (3.3593, -4.4997)
  line L2243 (0.0223, -5.5055) -> (0.0454, -5.5378)
  line L2244 (0.0013, -5.4717) -> (0.0223, -5.5055)
  line L2245 (-0.0478, -5.3633) -> (-0.0338, -5.4005)
  line L2246 (-0.0748, -5.2474) -> (-0.0683, -5.2866)
  line L2247 (-0.0593, -5.3253) -> (-0.0478, -5.3633)
  line L2248 (-0.0174, -5.4367) -> (0.0013, -5.4717)
  line L2249 (-0.0174, -5.4367) -> (0.0013, -5.4717)
  line L2250 (-0.0338, -5.4005) -> (-0.0174, -5.4367)
  line L2251 (-0.0683, -5.2866) -> (-0.0593, -5.3253)
  line L2252 (-0.0478, -5.3633) -> (-0.0338, -5.4005)
  line L2253 (6.02, -10.1995) -> (6.02, -12.839)
  line L2254 (19.8574, -5.4367) -> (19.8738, -5.4005)
  line L2255 (19.8738, -5.4005) -> (19.8878, -5.3633)
  line L2256 (13.82, -10.1995) -> (13.6201, -9.9997)
  line L2257 (19.9148, -5.2474) -> (19.9187, -5.2079)
  arc A145 (18.12, -6.7368) -> (18.4614, -6.8782) centre (18.32, -6.7368) ccw
  line L2258 (13.82, -12.839) -> (13.82, -10.1995)
  line L2259 (14.7514, 0.0003) -> (14.7117, -0.001)
  line L2260 (10.127, -6.0997) -> (9.92, -6.3044)
  line L2261 (12.7593, -6.0997) -> (10.127, -6.0997)
  line L2262 (19.9187, -5.2079) -> (19.92, -5.1682)
  line L2263 (19.9187, -5.2079) -> (19.92, -5.1682)
  circle A146 centre (9.92, -9.9997) radius 2.1
  line L2264 (9.7152, -6.0997) -> (7.0807, -6.0997)
  line L2265 (14.3222, -0.1775) -> (13.0414, -1.4582)
  line L2266 (9.7152, -6.0997) -> (7.0807, -6.0997)
  line L2267 (19.92, -5.1682) -> (19.92, -1.4997)
  line L2268 (18.12, -4.4997) -> (18.12, -6.7368)
  line L2269 (19.7694, -5.5685) -> (19.7946, -5.5378)
  line L2270 (18.12, -4.4997) -> (18.12, -6.7368)
  line L2271 (13.82, -7.1603) -> (16.4807, -4.4997)
  line L2272 (14.3222, -0.1775) -> (13.0414, -1.4582)
  line L2273 (19.8177, -5.5055) -> (19.8387, -5.4717)
  line L2274 (19.9083, -5.2866) -> (19.9148, -5.2474)
  line L2275 (19.8993, -5.3253) -> (19.9083, -5.2866)
  arc A147 (13.0414, -1.4582) -> (13.1828, -1.7997) centre (13.1828, -1.5997) ccw
  line L2276 (19.92, -1.4997) -> (19.92, -0.4997)
  line L2277 (10.127, -6.0997) -> (9.92, -6.3044)
  line L2278 (13.82, -12.839) -> (13.82, -10.1995)
  line L2279 (13.82, -9.7998) -> (13.82, -7.1603)
  circle A148 centre (9.92, -9.9997) radius 2.1
  line L2280 (13.6201, -9.9997) -> (13.82, -9.7998)
  line L2281 (13.82, -10.1995) -> (13.6201, -9.9997)
  line L2282 (19.7694, -5.5685) -> (19.7946, -5.5378)
  line L2283 (19.8387, -5.4717) -> (19.8574, -5.4367)
  line L2284 (19.7422, -5.5975) -> (19.7694, -5.5685)
  line L2285 (19.8574, -5.4367) -> (19.8738, -5.4005)
  line L2286 (15.42, -3.439) -> (12.7593, -6.0997)
  line L2287 (13.1828, -1.7997) -> (15.42, -1.7997)
  line L2288 (15.42, -3.439) -> (12.7593, -6.0997)
  line L2289 (14.4479, -0.081) -> (14.4142, -0.102)
  line L2290 (6.02, -10.1995) -> (6.02, -12.839)
  line L2291 (19.8738, -5.4005) -> (19.8878, -5.3633)
  line L2292 (19.9083, -5.2866) -> (19.9148, -5.2474)
  line L2293 (19.7946, -5.5378) -> (19.8177, -5.5055)
  arc A149 (19.92, -0.4997) -> (19.42, 0.0003) centre (19.42, -0.4997) ccw
  line L2294 (13.82, -9.7998) -> (13.82, -7.1603)
  line L2295 (13.82, -7.1603) -> (16.4807, -4.4997)
  line L2296 (14.5943, -0.0203) -> (14.5563, -0.0319)
  arc A150 (18.12, -6.7368) -> (18.4614, -6.8782) centre (18.32, -6.7368) ccw
  line L2297 (19.7946, -5.5378) -> (19.8177, -5.5055)
  line L2298 (19.8993, -5.3253) -> (19.9083, -5.2866)
  line L2299 (16.4807, -4.4997) -> (18.12, -4.4997)
  line L2300 (19.9148, -5.2474) -> (19.9187, -5.2079)
  line L2301 (19.7422, -5.5975) -> (19.7694, -5.5685)
  line L2302 (19.92, -5.1682) -> (19.92, -1.4997)
  line L2303 (14.5191, -0.0459) -> (14.483, -0.0623)
  line L2304 (14.483, -0.0623) -> (14.4479, -0.081)
  line L2305 (18.42, 0.0003) -> (14.7514, 0.0003)
  line L2306 (14.6722, -0.0049) -> (14.633, -0.0113)
  line L2307 (13.1828, -1.7997) -> (15.42, -1.7997)
  arc A151 (19.92, -0.4997) -> (19.42, 0.0003) centre (19.42, -0.4997) ccw
  line L2308 (18.4614, -6.8782) -> (19.7422, -5.5975)
  line L2309 (16.4807, -4.4997) -> (18.12, -4.4997)
  line L2310 (14.3819, -0.1251) -> (14.3512, -0.1503)
  line L2311 (19.42, 0.0003) -> (18.42, 0.0003)
  line L2312 (14.3512, -0.1503) -> (14.3222, -0.1775)
  line L2313 (14.4142, -0.102) -> (14.3819, -0.1251)
  line L2314 (14.3512, -0.1503) -> (14.3222, -0.1775)
  line L2315 (14.5943, -0.0203) -> (14.5563, -0.0319)
  line L2316 (15.42, -1.7997) -> (15.42, -3.439)
  line L2317 (14.5191, -0.0459) -> (14.483, -0.0623)
  line L2318 (14.7117, -0.001) -> (14.6722, -0.0049)
  line L2319 (14.7514, 0.0003) -> (14.7117, -0.001)
  line L2320 (19.92, -1.4997) -> (19.92, -0.4997)
  line L2321 (19.8387, -5.4717) -> (19.8574, -5.4367)
  line L2322 (14.633, -0.0113) -> (14.5943, -0.0203)
  line L2323 (14.7117, -0.001) -> (14.6722, -0.0049)
  line L2324 (19.8878, -5.3633) -> (19.8993, -5.3253)
  line L2325 (14.633, -0.0113) -> (14.5943, -0.0203)
  line L2326 (18.42, 0.0003) -> (14.7514, 0.0003)
  line L2327 (19.42, 0.0003) -> (18.42, 0.0003)
  line L2328 (14.6722, -0.0049) -> (14.633, -0.0113)
  line L2329 (14.5563, -0.0319) -> (14.5191, -0.0459)
  line L2330 (15.42, -1.7997) -> (15.42, -3.439)
  line L2331 (19.8177, -5.5055) -> (19.8387, -5.4717)
  line L2332 (18.4614, -6.8782) -> (19.7422, -5.5975)
  line L2333 (19.8878, -5.3633) -> (19.8993, -5.3253)
  line L2334 (14.5563, -0.0319) -> (14.5191, -0.0459)
  line L2335 (14.483, -0.0623) -> (14.4479, -0.081)
  line L2336 (14.4479, -0.081) -> (14.4142, -0.102)
  line L2337 (14.4142, -0.102) -> (14.3819, -0.1251)
  line L2338 (14.3819, -0.1251) -> (14.3512, -0.1503)
  line L2339 (19.8387, -154.5276) -> (19.8177, -154.4938)
  line L2340 (19.8177, -154.4938) -> (19.7946, -154.4616)
  line L2341 (19.8574, -154.5626) -> (19.8387, -154.5276)
  line L2342 (19.8738, -154.5988) -> (19.8574, -154.5626)
  line L2343 (19.8878, -154.636) -> (19.8738, -154.5988)
  arc A152 (18.4614, -153.1211) -> (18.12, -153.2625) centre (18.32, -153.2625) ccw
  line L2344 (19.9083, -154.7127) -> (19.8993, -154.674)
  line L2345 (19.7694, -154.4308) -> (19.7422, -154.4019)
  line L2346 (19.8993, -154.674) -> (19.8878, -154.636)
  line L2347 (19.7422, -154.4019) -> (18.4614, -153.1211)
  line L2348 (19.8177, -154.4938) -> (19.7946, -154.4616)
  arc A153 (18.4614, -153.1211) -> (18.12, -153.2625) centre (18.32, -153.2625) ccw
  line L2349 (19.9148, -154.7519) -> (19.9083, -154.7127)
  line L2350 (19.7694, -154.4308) -> (19.7422, -154.4019)
  line L2351 (19.7946, -154.4616) -> (19.7694, -154.4308)
  line L2352 (19.9187, -145.2079) -> (19.92, -145.1682)
  line L2353 (19.7694, -145.5685) -> (19.7946, -145.5378)
  line L2354 (18.4614, -146.8782) -> (19.7422, -145.5975)
  line L2355 (15.42, -143.439) -> (12.7593, -146.0997)
  line L2356 (13.1828, -141.7997) -> (15.42, -141.7997)
  line L2357 (19.9187, -145.2079) -> (19.92, -145.1682)
  line L2358 (19.8993, -145.3253) -> (19.9083, -145.2866)
  line L2359 (6.02, -110.1995) -> (6.02, -112.839)
  line L2360 (14.3222, -140.1775) -> (13.0414, -141.4582)
  line L2361 (18.4614, -146.8782) -> (19.7422, -145.5975)
  line L2362 (13.1828, -141.7997) -> (15.42, -141.7997)
  line L2363 (19.9148, -145.2474) -> (19.9187, -145.2079)
  line L2364 (19.8177, -145.5055) -> (19.8387, -145.4717)
  line L2365 (15.42, -143.439) -> (12.7593, -146.0997)
  line L2366 (19.92, -145.1682) -> (19.92, -141.4997)
  line L2367 (19.8878, -145.3633) -> (19.8993, -145.3253)
  line L2368 (19.9083, -145.2866) -> (19.9148, -145.2474)
  line L2369 (14.3222, -140.1775) -> (13.0414, -141.4582)
  line L2370 (19.8387, -145.4717) -> (19.8574, -145.4367)
  line L2371 (19.92, -145.1682) -> (19.92, -141.4997)
  line L2372 (19.9148, -145.2474) -> (19.9187, -145.2079)
  line L2373 (19.8387, -145.4717) -> (19.8574, -145.4367)
  line L2374 (19.92, -141.4997) -> (19.92, -140.4997)
  line L2375 (19.92, -141.4997) -> (19.92, -140.4997)
  line L2376 (6.02, -147.1603) -> (6.02, -149.7998)
  line L2377 (-0.0683, -154.7127) -> (-0.0748, -154.7519)
  line L2378 (1.3786, -153.1211) -> (0.0978, -154.4019)
  line L2379 (6.2199, -149.9997) -> (6.02, -150.1995)
  line L2380 (6.02, -149.7998) -> (6.2199, -149.9997)
  line L2381 (6.02, -147.1603) -> (6.02, -149.7998)
  line L2382 (9.7152, -146.0997) -> (7.0807, -146.0997)
  line L2383 (9.7152, -146.0997) -> (7.0807, -146.0997)
  line L2384 (6.02, -149.7998) -> (6.2199, -149.9997)
  line L2385 (6.2199, -149.9997) -> (6.02, -150.1995)
  line L2386 (-0.0593, -154.674) -> (-0.0683, -154.7127)
  line L2387 (-0.0338, -154.5988) -> (-0.0478, -154.636)
  line L2388 (-0.0748, -154.7519) -> (-0.0787, -154.7914)
  arc A154 (1.72, -153.2625) -> (1.3786, -153.1211) centre (1.52, -153.2625) ccw
  line L2389 (0.0223, -154.4938) -> (0.0013, -154.5276)
  line L2390 (-0.0593, -154.674) -> (-0.0683, -154.7127)
  line L2391 (-0.0478, -154.636) -> (-0.0593, -154.674)
  line L2392 (0.0013, -154.5276) -> (-0.0174, -154.5626)
  line L2393 (-0.0683, -154.7127) -> (-0.0748, -154.7519)
  line L2394 (0.0978, -154.4019) -> (0.0706, -154.4308)
  line L2395 (-0.0174, -154.5626) -> (-0.0338, -154.5988)
  line L2396 (0.0223, -154.4938) -> (0.0013, -154.5276)
  line L2397 (0.0978, -154.4019) -> (0.0706, -154.4308)
  line L2398 (-0.0478, -154.636) -> (-0.0593, -154.674)
  line L2399 (-0.0748, -154.7519) -> (-0.0787, -154.7914)
  line L2400 (0.0706, -154.4308) -> (0.0454, -154.4616)
  line L2401 (0.0454, -154.4616) -> (0.0223, -154.4938)
  line L2402 (1.72, -157.2997) -> (3.6807, -157.2997)
  line L2403 (6.02, -150.1995) -> (6.02, -152.839)
  line L2404 (-0.0338, -154.5988) -> (-0.0478, -154.636)
  line L2405 (1.72, -157.2997) -> (3.6807, -157.2997)
  line L2406 (-0.0174, -154.5626) -> (-0.0338, -154.5988)
  arc A155 (1.72, -153.2625) -> (1.3786, -153.1211) centre (1.52, -153.2625) ccw
  line L2407 (0.0706, -154.4308) -> (0.0454, -154.4616)
  line L2408 (-0.0787, -154.7914) -> (-0.08, -154.8997)
  line L2409 (0.0454, -154.4616) -> (0.0223, -154.4938)
  line L2410 (1.3786, -153.1211) -> (0.0978, -154.4019)
  line L2411 (3.3593, -155.4997) -> (1.72, -155.4997)
  line L2412 (0.0013, -154.5276) -> (-0.0174, -154.5626)
  line L2413 (6.02, -150.1995) -> (6.02, -152.839)
  line L2414 (3.3593, -155.4997) -> (1.72, -155.4997)
  line L2415 (1.72, -155.4997) -> (1.72, -153.2625)
  line L2416 (3.6807, -157.2997) -> (7.0807, -153.8997)
  line L2417 (6.02, -152.839) -> (3.3593, -155.4997)
  line L2418 (1.72, -155.4997) -> (1.72, -153.2625)
  line L2419 (3.6807, -157.2997) -> (7.0807, -153.8997)
  line L2420 (6.02, -152.839) -> (3.3593, -155.4997)
  line L2421 (-0.0787, -154.7914) -> (-0.08, -154.8997)
  line L2422 (13.82, -149.7998) -> (13.82, -147.1603)
  line L2423 (13.82, -152.839) -> (13.82, -150.1995)
  line L2424 (9.92, -153.6927) -> (10.127, -153.8997)
  line L2425 (10.127, -153.8997) -> (12.7593, -153.8997)
  line L2426 (13.82, -150.1995) -> (13.6201, -149.9997)
  line L2427 (9.713, -153.8997) -> (9.92, -153.6927)
  line L2428 (9.92, -153.6927) -> (10.127, -153.8997)
  circle A156 centre (9.92, -149.9997) radius 2.1
  line L2429 (13.6201, -149.9997) -> (13.82, -149.7998)
  line L2430 (10.127, -153.8997) -> (12.7593, -153.8997)
  line L2431 (13.82, -150.1995) -> (13.6201, -149.9997)
  line L2432 (9.713, -153.8997) -> (9.92, -153.6927)
  circle A157 centre (9.92, -149.9997) radius 2.1
  line L2433 (13.82, -152.839) -> (13.82, -150.1995)
  line L2434 (13.6201, -149.9997) -> (13.82, -149.7998)
  line L2435 (13.82, -149.7998) -> (13.82, -147.1603)
  line L2436 (19.9198, -5.7004) -> (19.9533, -5.6596)
  line L2437 (19.9533, -5.6596) -> (19.9841, -5.6166)
  line L2438 (19.9841, -5.6166) -> (20.012, -5.5718)
  line L2439 (20.012, -5.5718) -> (20.0369, -5.5252)
  line L2440 (20.0369, -5.5252) -> (20.0587, -5.4771)
  line L2441 (20.0587, -5.4771) -> (20.0773, -5.4277)
  line L2442 (20.0773, -5.4277) -> (20.0926, -5.3771)
  line L2443 (20.0926, -5.3771) -> (20.1046, -5.3257)
  line L2444 (20.1046, -5.3257) -> (20.1132, -5.2736)
  line L2445 (20.1132, -5.2736) -> (20.1184, -5.221)
  line L2446 (20.1184, -5.221) -> (20.12, -5.1715)
  line L2447 (20.12, -5.1715) -> (20.12, -1.4997)
  line L2448 (20.12, -1.4997) -> (20.12, -0.4997)
  arc A158 (20.12, -0.4997) -> (19.42, 0.2003) centre (19.42, -0.4997) ccw
  line L2449 (19.42, 0.2003) -> (18.42, 0.2003)
  line L2450 (18.42, 0.2003) -> (14.7482, 0.2003)
  line L2451 (14.7482, 0.2003) -> (14.6987, 0.1987)
  line L2452 (14.6987, 0.1987) -> (14.6461, 0.1935)
  line L2453 (14.6461, 0.1935) -> (14.594, 0.1849)
  line L2454 (14.594, 0.1849) -> (14.5425, 0.1729)
  line L2455 (14.5425, 0.1729) -> (14.492, 0.1576)
  line L2456 (14.492, 0.1576) -> (14.4426, 0.139)
  line L2457 (14.4426, 0.139) -> (14.3945, 0.1172)
  line L2458 (14.3945, 0.1172) -> (14.3479, 0.0923)
  line L2459 (14.3479, 0.0923) -> (14.303, 0.0644)
  line L2460 (14.303, 0.0644) -> (14.2601, 0.0337)
  line L2461 (14.2601, 0.0337) -> (14.2193, 0.0001)
  line L2462 (14.2193, 0.0001) -> (14.1831, -0.0337)
  line L2463 (14.1831, -0.0337) -> (12.9, -1.3168)
  arc A159 (12.9, -1.3168) -> (13.1828, -1.9997) centre (13.1828, -1.5997) ccw
  line L2464 (13.1828, -1.9997) -> (15.22, -1.9997)
  line L2465 (15.22, -1.9997) -> (15.22, -3.3562)
  line L2466 (15.22, -3.3562) -> (12.6765, -5.8997)
  line L2467 (12.6765, -5.8997) -> (10.0448, -5.8997)
  line L2468 (10.0448, -5.8997) -> (9.9208, -6.0223)
  line L2469 (9.9208, -6.0223) -> (9.7981, -5.8997)
  line L2470 (9.7981, -5.8997) -> (7.1635, -5.8997)
  line L2471 (7.1635, -5.8997) -> (4.62, -3.3562)
  line L2472 (4.62, -3.3562) -> (4.62, -1.9997)
  line L2473 (4.62, -1.9997) -> (6.6572, -1.9997)
  arc A160 (6.6572, -1.9997) -> (6.94, -1.3168) centre (6.6572, -1.5997) ccw
  line L2474 (6.94, -1.3168) -> (5.6569, -0.0337)
  line L2475 (5.6569, -0.0337) -> (5.6207, 0.0001)
  line L2476 (5.6207, 0.0001) -> (5.5799, 0.0337)
  line L2477 (5.5799, 0.0337) -> (5.537, 0.0644)
  line L2478 (5.537, 0.0644) -> (5.4921, 0.0923)
  line L2479 (5.4921, 0.0923) -> (5.4455, 0.1172)
  line L2480 (5.4455, 0.1172) -> (5.3974, 0.139)
  line L2481 (5.3974, 0.139) -> (5.348, 0.1576)
  line L2482 (5.348, 0.1576) -> (5.2975, 0.1729)
  line L2483 (5.2975, 0.1729) -> (5.246, 0.1849)
  line L2484 (5.246, 0.1849) -> (5.1939, 0.1935)
  line L2485 (5.1939, 0.1935) -> (5.1413, 0.1987)
  line L2486 (5.1413, 0.1987) -> (5.0918, 0.2003)
  line L2487 (5.0918, 0.2003) -> (1.42, 0.2003)
  line L2488 (1.42, 0.2003) -> (0.42, 0.2003)
  arc A161 (0.42, 0.2003) -> (-0.28, -0.4997) centre (0.42, -0.4997) ccw
  line L2489 (-0.28, -0.4997) -> (-0.28, -1.4997)
  line L2490 (-0.28, -1.4997) -> (-0.28, -5.1009)
  line L2491 (-0.28, -5.1009) -> (-0.2786, -5.2189)
  line L2492 (-0.2786, -5.2189) -> (-0.2732, -5.2736)
  line L2493 (-0.2732, -5.2736) -> (-0.2646, -5.3257)
  line L2494 (-0.2646, -5.3257) -> (-0.2526, -5.3771)
  line L2495 (-0.2526, -5.3771) -> (-0.2373, -5.4277)
  line L2496 (-0.2373, -5.4277) -> (-0.2187, -5.4771)
  line L2497 (-0.2187, -5.4771) -> (-0.1969, -5.5252)
  line L2498 (-0.1969, -5.5252) -> (-0.172, -5.5718)
  line L2499 (-0.172, -5.5718) -> (-0.1441, -5.6166)
  line L2500 (-0.1441, -5.6166) -> (-0.1133, -5.6596)
  line L2501 (-0.1133, -5.6596) -> (-0.0798, -5.7004)
  line L2502 (-0.0798, -5.7004) -> (-0.0459, -5.7366)
  line L2503 (-0.0459, -5.7366) -> (1.2372, -7.0197)
  arc A162 (1.2372, -7.0197) -> (1.92, -6.7368) centre (1.52, -6.7368) ccw
  line L2504 (1.92, -6.7368) -> (1.92, -4.6997)
  line L2505 (1.92, -4.6997) -> (3.2765, -4.6997)
  line L2506 (3.2765, -4.6997) -> (5.82, -7.2432)
  line L2507 (5.82, -7.2432) -> (5.82, -9.8826)
  line L2508 (5.82, -9.8826) -> (5.937, -9.9997)
  line L2509 (5.937, -9.9997) -> (5.82, -10.1167)
  line L2510 (5.82, -10.1167) -> (5.82, -12.7562)
  line L2511 (5.82, -12.7562) -> (3.2765, -15.2997)
  line L2512 (3.2765, -15.2997) -> (1.92, -15.2997)